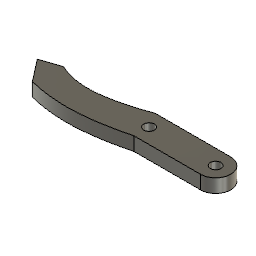
Gripper Holder 3.0 (Autodesk Fusion 360 design; units mm, degrees)
part number: 2026-08-19-22-23-44-975
Autodesk Fusion 360 part; units mm, degrees
sketch "Sketch1" plane through (0, 0, 0) normal (0, 0, 1) x (1, 0, 0)
  line L0 (-11, 0) -> (11, 0) construction
  circle A0 centre (-11, 0) radius 1.75
  circle A1 centre (-11, 0) radius 5
  circle A2 centre (11, 0) radius 1.75
  circle A3 centre (11, 0) radius 5
  line L1 (-11, 5) -> (11, 5)
  line L2 (11, -5) -> (-11, -5)
  dimension "d1" = 22
  dimension "d2" = 3.5
  dimension "d3" = 10
  dimension "d4" = 3.5
  dimension "d5" = 10
  constraint midpoint L0 origin
  constraint horizontal L0
  constraint coincident L0.start A0.centre
  constraint concentric A0 A1
  constraint coincident L0.end A2.centre
  constraint concentric A2 A3
  constraint coincident A1 L1.start
  constraint coincident A3 L1.end
  constraint tangent A3 L1
  constraint coincident A3 L2.start
  constraint coincident A1 L2.end
  constraint tangent A1 L2
  measures "d1" distance of L0.start L0.end
  measures "d2" diameter of A0
  measures "d3" diameter of A1
  measures "d4" diameter of A2
  measures "d5" diameter of A3
extrude "Extrude1" add sketch "Sketch1" along normal blind 4.5
sketch "Sketch2" plane through (0, 0, 4.5) normal (0, 0, 1) x (-1, 0, 0)
  circle A0 centre (-11, 0) radius 1.75
  circle A1 centre (11, 0) radius 1.75
  arc A2 (11, -5) -> (11, 5) centre (11, 0) ccw
  line L0 (11, 5) -> (-11, 5)
  arc A3 (-11, 5) -> (-11, -5) centre (-11, 0) ccw
  line L1 (-11, -5) -> (11, -5)
  line L2 (11, 0) -> (11, -5) construction
  line L3 (0, 0) -> (0, 5) construction
  line L4 (11, 0) -> (11, 5) construction
  line L5 (0, 5) -> (11, 5)
  line L6 (13.99, -5) -> (11, -5)
  line L7 (13.99, -5) -> (11, -5)
  line L8 (13.99, -5) -> (11, -5)
  line L9 (0, 4.95) -> (0, 5.05)
  spline S0 degree 5 poles (43.3827, 6.2519) (42.8142, 6.3943) (41.6699, 6.6641) (39.9322, 7.0237) (37.572, 7.4115) (34.5449, 7.7335) (31.4348, 7.8797) (28.2359, 7.8379) (24.947, 7.6056) (21.5738, 7.1946) (18.1233, 6.6201) (15.3067, 6.0413) (13.1647, 5.5446) (11.7237, 5.1861) (11, 5) knots 0 0 0 0 0 0 0.1 0.2 0.3 0.4 0.5 0.6 0.7 0.8 0.9 1 1 1 1 1 1
  line L10 (49, -1) -> (43.3827, 6.2519)
  circle A4 centre (11, 0) radius 5
  line L11 (49, -1) -> (42.4735, -3.2067)
  spline S1 degree 5 poles (13.99, -5) (14.3125, -4.8777) (14.9644, -4.6352) (15.9628, -4.2778) (17.3358, -3.8142) (19.1224, -3.2581) (20.9787, -2.73) (22.901, -2.2385) (24.8802, -1.7975) (26.9002, -1.4266) (28.9415, -1.1487) (30.9832, -0.9869) (33.006, -0.962) (34.9943, -1.0892) (36.9392, -1.3746) (38.8366, -1.8183) (40.3155, -2.2977) (41.4029, -2.7258) (42.1182, -3.0414) (42.4735, -3.2067) knots 0 0 0 0 0 0 0.066667 0.133333 0.2 0.266667 0.333333 0.4 0.466667 0.533333 0.6 0.666667 0.733333 0.8 0.866667 0.933333 1 1 1 1 1 1
  point P0 (0, 5)
  point P1 (0, 5)
  point P2 (29.1574, 7.8223)
  point P3 (22.5528, -2.3387)
  point P4 (33, -1)
  dimension "d18" = 2.99
  dimension "d27" = 2.99
  dimension "d28" = 2.99
  constraint coincident A1.centre A2.centre
  constraint coincident A2.start L1.end
  constraint coincident L3.start origin
  constraint midpoint L0 P1
  constraint coincident A2.end L0.start
  constraint tangent A2 L6
  constraint coincident P1 P0
  constraint midpoint P1 L9
  constraint perpendicular L5 L9
  measures "d18" distance of A2.start L6.start
  measures "d27" distance of A2.start L6.start
  measures "d28" distance of A2.start L6.start
extrude "Extrude3" add sketch "Sketch2" against normal up to surface (4.5 mm away) contours A2 L6 L7 L8 S0 L10 A4 L11 S1
extrude "Extrude2" [suppressed]
